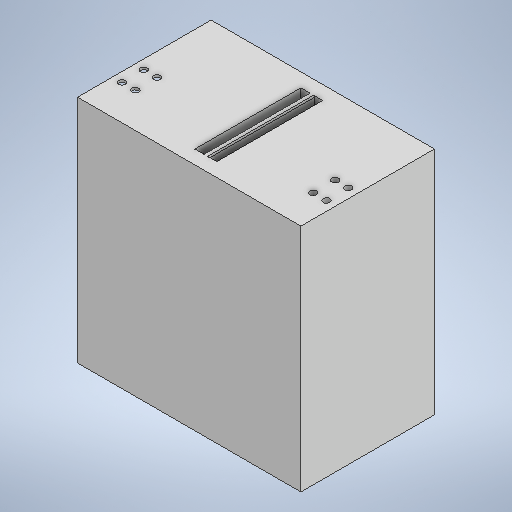
# Autodesk Inventor part: obudowa_silnik_H100_L11_W56
Saved by Autodesk Inventor 2025.2 (Build 292293000, 293)
## iProperties
Created: 2025-03-20
Part Number: obudowa_silnik_H100_L11_W56
Material: Ogólny
Document SubType Name: Modeling
Designer: rango
Density: 1 g/cm^3
Appearance: Domyślna
Author: rango
Autodesk Inventor part; units mm, degrees
ref_plane "YZ Plane" through (0, 0, 0) normal (1, 0, 0) x (0, 1, 0)
ref_plane "XZ Plane" through (0, 0, 0) normal (0, 1, 0) x (-1, 0, 0)
ref_plane "XY Plane" through (0, 0, 0) normal (0, 0, 1) x (1, 0, 0)
sketch "Szkic1" plane through (0, 0, 0) normal (1, 0, 0) x (0, 1, 0)
  line L0 (29, 29) -> (-29, 29)
  line L1 (-29, 29) -> (-29, -29)
  line L2 (-29, -29) -> (29, -29)
  line L3 (29, -29) -> (29, 29)
  line L4 (28, 28) -> (-28, 28)
  line L5 (-28, 28) -> (-28, -28)
  line L6 (-28, -28) -> (28, -28)
  line L7 (28, -28) -> (28, 28)
  point P0 (0, 0)
  dimension "d0" = 58
  dimension "d1" = 58
  dimension "d2" = 56
  dimension "d3" = 56
  constraints: 16 end point, 4 parallel, 2 horizontal, 2 perpendicular
  measures "d0" distance of L2.end L1.end
  measures "d1" distance of L1.end L0.end
  measures "d2" distance of L6.end L5.end
  measures "d3" distance of L5.end L4.end
extrude "Wyciągnięcie proste1" add sketch "Szkic1" along normal blind 56
sketch "Szkic2" plane through (56, 0, 0) normal (1, 0, 0) x (0, 0, -1)
  line L0 (29, 29) -> (-29, 29) projected
  line L1 (29, -29) -> (29, 29) projected
  line L2 (-29, 29) -> (29, 29)
  line L3 (29, 29) -> (29, -29)
  line L4 (29, -29) -> (-29, -29)
  line L5 (-29, -29) -> (-29, 29)
  point P0 (0, 0)
  constraints: 8 end point, 2 parallel, 1 horizontal, 1 perpendicular
extrude "Wyciągnięcie proste2" add sketch "Szkic2" along normal blind 2
sketch "Szkic3" plane through (0, 0, 0) normal (-1, 0, 0) x (0, 0, 1)
  line L0 (29, 50) -> (-29, 50)
  line L1 (-29, 50) -> (-29, -50)
  line L2 (-29, -50) -> (29, -50)
  line L3 (29, -50) -> (29, 50)
  line L4 (-28, 49) -> (28, 49)
  line L5 (28, 49) -> (28, -49)
  line L6 (28, -49) -> (-28, -49)
  line L7 (-28, -49) -> (-28, 49)
  point P0 (0, 0)
  dimension "d8" = 100
  dimension "d9" = 98
  constraints: 16 end point, 4 parallel, 2 horizontal, 2 perpendicular
  measures "d8" distance of L1.end L0.end
  measures "d9" distance of L4.end L5.end
extrude "Wyciągnięcie proste3" add sketch "Szkic3" along normal blind 50
sketch "Szkic4" plane through (0, 0, 0) normal (1, 0, 0) x (0, 0, -1)
  line L0 (-29, 29) -> (-29, 50) projected
  line L1 (29, -29) -> (29, 29) projected
  line L2 (-29, 50) -> (29, 50)
  line L3 (29, 50) -> (29, 29)
  line L4 (29, 29) -> (-29, 29)
  line L5 (-29, 29) -> (-29, 50)
  line L6 (29, -50) -> (-29, -50) projected
  line L7 (-29, -29) -> (29, -29)
  line L8 (29, -29) -> (29, -50)
  line L9 (29, -50) -> (-29, -50)
  line L10 (-29, -50) -> (-29, -29)
  point P0 (0, 0)
  constraints: 16 end point, 4 parallel, 2 horizontal, 2 perpendicular, 1 point on line
extrude "Wyciągnięcie proste4" add sketch "Szkic4" along normal blind 1
sketch "Szkic5" plane through (58, -29, -29) normal (0, 0, -1) x (-1, 0, 0)
  line L0 (108, 78) -> (108, -20) projected
  line L1 (58, 57) -> (108, 57)
  line L2 (108, 57) -> (108, 0.6199)
  line L3 (108, 0.6199) -> (58, 0.6199)
  line L4 (58, 0.6199) -> (58, 57)
  point P0 (58, 29)
  constraints: 8 end point, 2 parallel, 1 horizontal, 1 perpendicular, 1 point on line
extrude "Wyciągnięcie proste5" cut sketch "Szkic5" against normal blind 1
sketch "Szkic6" plane through (58, -29, -29) normal (0, 0, -1) x (-1, 0, 0)
  line L0 (108, 57) -> (58, 57) projected
  line L1 (83, 57) -> (83, 78)
  line L2 (58, 78) -> (108, 78) projected
  line L3 (108, 57) -> (108, 78) projected
  line L4 (108, 67.5) -> (57, 67.5)
  line L5 (57, 58) -> (57, 79) projected
  line L6 (58, -20) -> (108, -20) projected
  line L7 (83, -20) -> (83, 0.6199)
  line L8 (58, 0.6199) -> (108, 0.6199) projected
  line L9 (58, -20) -> (58, 1) projected
  line L10 (58, -9.5) -> (108, -9.5)
  line L11 (108, 0.6199) -> (108, -21) projected
  circle A0 centre (83, 67.5) radius 1.5
  circle A1 centre (83, -9.5) radius 1.5
  point P0 (58, 29)
  dimension "d16" = 3
  dimension "d17" = 3
  constraints: 8 end point, 8 midpoint, 3 point on line, 2 centre point, 2 perpendicular
  measures "d16" diameter of A0
  measures "d17" diameter of A1
hole "Otwór1" at (-25, 38.5, -29) at (-25, -38.5, -29) direction (0, 0, 1) diameter 4.9784 depth 1 tip angle 118 thread size "1/4-20 UNC" class "2B" standard "ANSI Unified Screw Threads"
sketch "Szkic7" plane through (58, -29, 29) normal (0, 0, 1) x (1, 0, 0)
  line L0 (-57, 79) -> (-57, 58) projected
  line L1 (-57, 79) -> (0, 79)
  line L2 (0, 58) -> (0, 0) projected
  line L3 (0, 79) -> (0, 58)
  line L4 (-57, -21) -> (-108, -21) projected
  line L5 (-57, -21) -> (0, -21)
  line L6 (0, -21) -> (0, 0)
  line L7 (-57, 58) -> (0, 58) projected
  line L8 (0, 58) -> (-57, 58)
  line L9 (-57, 58) -> (-57, 79)
  line L10 (-57, -21) -> (-57, 0)
  line L11 (-57, 0) -> (0, 0)
  point P0 (-58, 29)
  constraints: 16 end point, 4 perpendicular, 2 collinear, 1 horizontal, 1 point on line
extrude "Wyciągnięcie proste6" add sketch "Szkic7" against normal blind 58
sketch "Szkic8" plane through (58, 50, -29) normal (0, 0, -1) x (-1, 0, 0)
  line L0 (0, 0) -> (108, 0) projected
  line L1 (108, 0) -> (97, 0)
  line L2 (97, 0) -> (97, -100)
  line L3 (0, -100) -> (108, -100) projected
  line L4 (108, -100) -> (97, -100)
  line L5 (108, -100) -> (108, 0)
  line L6 (97, 0) -> (108, 0)
  point P0 (58, -50)
  dimension "d27" = 11
  constraints: 10 end point, 2 perpendicular, 2 point on line, 1 collinear, 1 vertical
  measures "d27" distance of L0.end L1.end
extrude "Wyciągnięcie proste7" cut sketch "Szkic8" against normal blind 58
sketch "Szkic9" plane through (58, -50, -29) normal (0, -1, 0) x (1, 0, 0)
  line L0 (0, 58) -> (-97, 58) projected
  line L1 (-97, 0) -> (-97, 58) projected
  line L2 (-92.9215, 33.311) -> (-92.9215, 42.811)
  line L3 (0, 0) -> (-97, 0) projected
  line L4 (-87.1435, 33.311) -> (-97, 33.311)
  line L5 (-87.1435, 33.311) -> (-87.1435, 42.811)
  line L6 (-87.1435, 42.811) -> (-92.9215, 42.811)
  line L7 (-92.9215, 42.811) -> (-92.9215, 33.311)
  line L8 (-97, 0) -> (-48.5, 0)
  line L9 (0, 58) -> (0, 0) projected
  point P0 (-9.857, 42.811)
  point P1 (-9.857, 33.311)
  point P2 (-4.079, 33.311)
  point P3 (-4.079, 42.811)
  dimension "d54" = 5.778
  dimension "d59" = 5.778
  dimension "d60" = 33.311
  dimension "d61" = 9.5
  dimension "d68" = 4.0785
  dimension "d70" = 9.5
  dimension "d71" = 9.5
  dimension "d72" = 5.778
  dimension "d73" = 5.778
  dimension "d74" = 4.079
  dimension "d75" = 77.2865
  dimension "d76" = 77.2865
  constraints: 12 end point, 2 perpendicular, 2 vertical, 1 horizontal, 1 midpoint, 1 point on line
  measures "d54" distance of L4.start L2.start
  measures "d59" distance of L2.end L5.end
  measures "d60" distance from line of L4.start L3
  measures "d61" distance of L4.start L5.end
  measures "d68" distance between parallel lines of L1 L2
  measures "d70" distance of point (-9.857, 42.811) point (-9.857, 33.311)
  measures "d71" distance of point (-4.079, 42.811) point (-4.079, 33.311)
  measures "d72" distance of point (-9.857, 33.311) point (-4.079, 33.311)
  measures "d73" distance of point (-4.079, 42.811) point (-9.857, 42.811)
  measures "d74" distance from line of L9 point (-4.079, 42.811)
  measures "d75" distance of L5.end point (-9.857, 42.811)
  measures "d76" distance of L4.start point (-9.857, 33.311)
hole "Otwór2" at (-29.1435, -50, 4.311) at (-29.1435, -50, 13.811) at (-34.9215, -50, 4.311) at (-34.9215, -50, 13.811) at (48.143, -50, 13.811) at (53.921, -50, 13.811) at (53.921, -50, 4.311) at (48.143, -50, 4.311) direction (0, 1, 0) diameter 3 end through all
sketch "Szkic10" plane through (58, 50, 29) normal (0, 1, 0) x (1, 0, 0)
  line L0 (0, 0) -> (-97, 0)
  line L1 (-58, 1) -> (-97, 1) projected
  line L2 (0, 58) -> (-97, 58) projected
  line L3 (-97, 0) -> (-97, 58)
  line L4 (-97, 58) -> (0, 58)
  line L5 (0, 58) -> (0, 0)
  line L6 (-58, 1) -> (-2, 1) projected
  line L7 (-48.5, 1) -> (-48.5, 58)
  line L8 (-48.5, 58) -> (-53.5, 58)
  line L9 (-53.5, 58) -> (-54.5822, 58)
  line L10 (-48.5, 58) -> (-53.5, 58)
  line L11 (-48.5, 58) -> (-51, 58)
  line L12 (-48.5, 1) -> (-46, 1)
  line L13 (-46, 1) -> (-46, 58)
  line L14 (-46, 1) -> (-46, 0)
  line L15 (-48.5, 1) -> (-48.5, 0)
  line L16 (-48.5, 58) -> (-46, 58)
  line L17 (-46, 0) -> (-42.5, 0)
  line L18 (-42.5, 0) -> (-42.5, 58)
  line L19 (-48.5, 58) -> (-52, 58)
  line L20 (-52, 58) -> (-52, 0)
  line L21 (-48.5, 0) -> (-52, 0)
  line L22 (-52, 58) -> (-52, 52)
  line L23 (-52, 52) -> (-42.5, 52)
  line L24 (-52, 0) -> (-52, 6)
  line L25 (-52, 6) -> (-42.5, 6)
  point P0 (-58, 29)
  point P1 (-46, 6)
  point P2 (-46, 52)
  point P3 (-48.5, 6)
  point P4 (-48.5, 52)
  dimension "d78" = 2.5
  dimension "d79" = 3.5
  dimension "d80" = 3.5
  dimension "d81" = 6
  dimension "d82" = 6
  constraints: 46 end point, 14 point on line, 9 perpendicular, 3 collinear, 3 midpoint, 1 parallel
  measures "d78" distance of L7.start L12.end
  measures "d79" distance of L14.end L17.end
  measures "d80" distance of L7.end L19.end
  measures "d81" distance of L19.end L22.end
  measures "d82" distance of L20.end L24.end
extrude "Wyciągnięcie proste8" cut sketch "Szkic10" against normal blind 17.5 contours L25 L13 L23 L18 | L25 L20 L23 L7
sketch "Szkic11" plane through (15.5, 50, -23) normal (-1, 0, 0) x (0, 0, 1)
  line L0 (0, -17.5) -> (46, -17.5) projected
  line L1 (46, -17.5) -> (46, -12.5)
  line L2 (46, 0) -> (46, -17.5) projected
  line L3 (46, -12.5) -> (0, -12.5)
  line L4 (0, 0) -> (0, -17.5) projected
  line L5 (0, -17.5) -> (46, -17.5)
  line L6 (0, -17.5) -> (0, -12.5)
  line L7 (46, -12.5) -> (46, -17.5)
  point P0 (23, -50)
  dimension "d85" = 5
  constraints: 10 end point, 2 equal length, 2 perpendicular, 2 point on line
  measures "d85" distance of L0.end L1.end
extrude "Wyciągnięcie proste9" cut sketch "Szkic11" along normal blind 9.75
fillet "Zaokrąglenie1" radius 0.5 2 edges at (9.5, 50, 0) (12, 50, 0)
